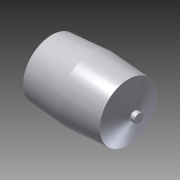
# Autodesk Inventor part: Kornylak- Roller
Saved by Autodesk Inventor 2014 (Build 180170000, 170)
## iProperties
Created: 2014-02-14
Part Number: Kornylak- Roller
Material: Generic
Document SubType Name: Modeling
Designer: Spooner
Density: 1 g/cm^3
Appearance: White
Mass: 0.659413 g
Surface Area: 4.04862 cm^2
Volume: 0.659413 cm^3
Author: Spooner
Autodesk Inventor part; units mm, degrees
ref_plane "YZ Plane" through (0, 0, 0) normal (1, 0, 0) x (0, 1, 0)
ref_plane "XZ Plane" through (0, 0, 0) normal (0, 1, 0) x (-1, 0, 0)
ref_plane "XY Plane" through (0, 0, 0) normal (0, 0, 1) x (1, 0, 0)
sketch "Sketch1" plane through (0, 0, 0) normal (0, 0, 1) x (1, 0, 0)
  line L0 (-6.985, 0) -> (-6.985, 0.635)
  line L1 (-6.985, 0.635) -> (-6.35, 0.635)
  line L2 (-6.35, 0.635) -> (-5.461, 4.064)
  line L3 (-5.461, 4.064) -> (0, 4.445)
  line L4 (0, 4.445) -> (5.461, 4.064)
  line L5 (5.461, 4.064) -> (6.35, 0.635)
  line L6 (6.35, 0.635) -> (6.985, 0.635)
  line L7 (6.985, 0.635) -> (6.985, 0)
  line L8 (6.985, 0) -> (-6.985, 0)
  point P0 (0, 0)
  point P1 (0, 0)
  dimension "d0" = 13.97
  dimension "d1" = 4.445
  dimension "d2" = 0.635
  dimension "d3" = 4.064
  dimension "d4" = 10.922
  dimension "d5" = 12.7
  constraints: 18 end point, 4 equal length, 2 parallel, 1 coincident, 1 collinear, 1 midpoint, 1 perpendicular, 1 vertical, 1 vertical alignment
  measures "d0" distance of L7.end L0.start
  measures "d1" distance from line of L3.end L8
  measures "d2" distance between parallel lines of L8 L1
  measures "d3" distance from line of L8 L2.end
  measures "d4" distance of L4.end L2.end
  measures "d5" distance of L5.end L1.end
revolve "Revolution1" add sketch "Sketch1" angle 360 about axis through (6.985, 0, 0) along (-1, 0, 0)
body "Solid1"
